Autodesk Fusion 360 part; units mm, degrees
note: some values were not read from the file. Chosen so that the rebuilt part matches the saved one: which face or edge a step refers to. Set by a fixed rule: which sketch regions a step uses.
(part 2 of 2)
copy_body "CopyPasteBodies18" bodies 51 52 makes body 53 makes body 54
move_body "Move24" bodies 53 54 to x (1, 0, 0) y (0, 1, 0) z (0, 0, 1) at (0, 0, 2.85)
copy_body "CopyPasteBodies19" bodies 51 52 53 54 makes body 55 makes body 56 makes body 57 makes body 58
move_body "Move25" bodies 55 56 57 58 to x (1, 0, 0) y (0, 1, 0) z (0, 0, 1) at (0, 0, 5)
copy_body "CopyPasteBodies20" bodies 51 52 53 54 55 56 57 58 makes body 59 makes body 60 makes body 61 makes body 62 makes body 63 makes body 64 makes body 65 makes body 66
move_body "Move26" bodies 59 60 61 62 63 64 65 66 to x (1, 0, 0) y (0, 1, 0) z (0, 0, 1) at (0, 0, -10.5)
move_body "Move27" bodies 58 57 to x (1, 0, 0) y (0, 1, 0) z (0, 0, 1) at (0, 0, -0.4)
extrude "Extrude25" add 1 faces at (5.7503, 0, 5.5348) along direction (0, -1, 0) blind 0.1 separate body on bodies 1 makes body 67
component "Component" placed x (1, 0, 0) y (0, 1, 0) z (0, 0, 1) at (0, 0, 0)
component "Component" placed x (1, 0, 0) y (0, 1, 0) z (0, 0, 1) at (7.1877, 0.1427, -14.6977)
component "Component''" placed x (1, 0, 0) y (0, 1, 0) z (0, 0, 1) at (0, 0, 0)
component "Component'''" placed x (1, 0, 0) y (0, 1, 0) z (0, 0, 1) at (0, 0, 0)
component "Component''''" placed x (1, 0, 0) y (0, 1, 0) z (0, 0, 1) at (0, 0, 0)
component "Component'''''" placed x (1, 0, 0) y (0, 1, 0) z (0, 0, 1) at (0, 0, 0)
component "Component''''''" placed x (1, 0, 0) y (0, 1, 0) z (0, 0, 1) at (0, 0, 0)
component "Component''" placed x (-1, 0, 0) y (0, 1, 0) z (0, 0, -1) at (-13.3695, 0, -0.2981)
component "Component'''''" placed x (-1, 0, 0) y (0, 1, 0) z (0, 0, -1) at (-13.3695, 0, -0.2981)
component "Component''''''" placed x (-1, 0, 0) y (0, 1, 0) z (0, 0, -1) at (-13.3695, 0, -0.2981)
component "Component'''" placed x (-1, 0, 0) y (0, 1, 0) z (0, 0, -1) at (-13.3695, 0, -0.2981)
component "Component''''" placed x (-1, 0, 0) y (0, 1, 0) z (0, 0, -1) at (-13.3695, 0, -0.2981)
component "Component''" placed x (-1, 0, 0) y (0, 1, 0) z (0, 0, -1) at (-26.8695, 0, 4.0019)
component "Component''" placed x (-1, 0, 0) y (0, 1, 0) z (0, 0, -1) at (-26.7695, 0, 9.1019)
component "Component''" placed x (-1, 0, 0) y (0, 1, 0) z (0, 0, -1) at (-26.7695, 0, 14.1019)
component "Component''''" placed x (0, 0, 1) y (0, 1, 0) z (-1, 0, 0) at (0.3833, -0.3, -9.2546)
component "Component''''" placed x (0, 0, 1) y (0, 1, 0) z (-1, 0, 0) at (0.3833, -0.3, -4.2546)
component "Component''''" placed x (0, 0, 1) y (0, 1, 0) z (-1, 0, 0) at (0.3833, -0.3, 0.4454)
component "Component'" placed x (1, 0, 0) y (0, 1, 0) z (0, 0, 1) at (0, 0, 0) in component "Component"
